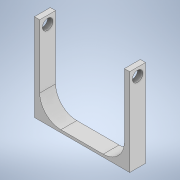
# Autodesk Inventor part: fork04
Saved by Autodesk Inventor 2021.2 (Build 252289000, 289)
## iProperties
Created: 2020-11-14
Part Number: fork04
Material: Generic
Document SubType Name: Modeling
Designer: robst
Density: 1 g/cm^3
Appearance: Default
Author: robst
Autodesk Inventor part; units mm, degrees
ref_plane "YZ Plane" through (0, 0, 0) normal (1, 0, 0) x (0, 1, 0)
ref_plane "XZ Plane" through (0, 0, 0) normal (0, 1, 0) x (-1, 0, 0)
ref_plane "XY Plane" through (0, 0, 0) normal (0, 0, 1) x (1, 0, 0)
sketch "Sketch1" plane through (0, 0, 0) normal (0, 1, 0) x (-1, 0, 0)
  line L0 (114.3, 19.05) -> (-114.3, 19.05)
  line L1 (-114.3, 19.05) -> (-114.3, -19.05)
  line L2 (-114.3, -19.05) -> (114.3, -19.05)
  line L3 (114.3, -19.05) -> (114.3, 19.05)
  line L4 (114.3, 19.05) -> (-114.3, -19.05) construction
  line L5 (-114.3, 19.05) -> (114.3, -19.05) construction
  point P0 (0, 0)
  dimension "d0" = 228.6
  dimension "d1" = 38.1
  constraints: 12 end point, 2 midpoint, 2 parallel, 1 horizontal, 1 perpendicular
  measures "d0" distance of L0.start L0.end
  measures "d1" distance of L1.end L0.end
extrude "Extrusion1" add sketch "Sketch1" against normal blind 6.35
sketch "Sketch2" plane through (0, 0, 0) normal (0, 1, 0) x (1, 0, 0)
  line L0 (-114.3, -19.05) -> (-114.3, 19.05) projected
  line L1 (-114.3, 19.05) -> (114.3, 19.05) projected
  line L2 (-114.3, -19.05) -> (-101.6, -19.05)
  line L3 (-101.6, -19.05) -> (-101.6, 19.05)
  line L4 (-101.6, 19.05) -> (-114.3, 19.05)
  line L5 (-114.3, 19.05) -> (-114.3, -19.05)
  line L6 (114.3, 19.05) -> (114.3, -19.05) projected
  line L7 (114.3, -19.05) -> (101.6, -19.05)
  line L8 (101.6, -19.05) -> (101.6, 19.05)
  line L9 (101.6, 19.05) -> (114.3, 19.05)
  line L10 (114.3, 19.05) -> (114.3, -19.05)
  point P0 (0, 0)
  dimension "d4" = 12.7
  dimension "d5" = 12.7
  constraints: 16 end point, 4 parallel, 2 horizontal, 2 perpendicular, 2 point on line
  measures "d4" distance between parallel lines of L3 L0
  measures "d5" distance between parallel lines of L6 L8
extrude "Extrusion2" add sketch "Sketch2" along normal blind 203.2
sketch "Sketch3" plane through (-114.3, -6.35, -19.05) normal (-1, 0, 0) x (0, 0, 1)
  line L0 (0, 209.55) -> (38.1, 209.55) construction
  line L1 (19.05, 209.55) -> (19.05, 0) construction
  line L2 (38.1, 0) -> (0, 0) construction
  circle A0 centre (19.05, 190.5) radius 12.7
  line L3 (0, 6.35) -> (0, 209.55) construction
  line L4 (0, 203.2) -> (38.1, 203.2) construction
  point P0 (19.05, 6.35)
  dimension "d8" = 25.4
  dimension "d9" = 6.35
  constraints: 4 end point, 2 midpoint, 2 point on line, 1 centre point, 1 horizontal, 1 tangent
  measures "d8" diameter of A0
  measures "d9" distance between parallel lines of L4 L0
extrude "Extrusion3" cut sketch "Sketch3" against normal through all
fillet "Fillet1" radius 50.8 2 edges at (101.6, 0, 0) (-101.6, 0, 0)
body "Solid1"
